Autodesk Fusion 360 part; units mm, degrees
(part 10 of 25)
  arc A1461 (56.8014, 41.9498) -> (56.508, 41.8283) centre (56.6547, 41.889) ccw
  line L369 (50.6695, 43.3959) -> (50.1845, 43.3959)
  line L370 (59.69, 41.0137) -> (59.96, 40.7437)
  arc A1462 (39.2664, 37.5968) -> (39.0418, 37.3723) centre (39.1541, 37.4846) ccw
  line L371 (42.1259, 37.4845) -> (42.1259, 37.9695)
  line L372 (52.2859, 41.2945) -> (52.2859, 41.7795)
  arc A1463 (50.9305, 40.5829) -> (50.9305, 40.2654) centre (50.9305, 40.4241) ccw
  arc A1464 (52.6557, 41.9247) -> (52.4312, 42.1493) centre (52.5434, 42.037) ccw
  arc A1465 (57.3078, 40.6314) -> (57.5323, 40.8559) centre (57.4201, 40.7437) ccw
  arc A1466 (43.5851, 43.6309) -> (43.5851, 43.3134) centre (43.5851, 43.4721) ccw
  line L373 (43.6534, 39.497) -> (49.7574, 39.497)
  arc A1467 (41.2555, 36.4554) -> (41.2555, 36.7728) centre (41.2555, 36.6141) ccw
  arc A1468 (39.9123, 36.5018) -> (40.1368, 36.7264) centre (40.0246, 36.6141) ccw
  line L374 (59.42, 40.7437) -> (59.69, 41.0137)
  arc A1469 (42.2846, 37.9695) -> (41.9671, 37.9695) centre (42.1258, 37.9695) ccw
  arc A1470 (58.0081, 40.3282) -> (58.1296, 40.6216) centre (58.0689, 40.4749) ccw
  line L375 (42.1259, 41.2945) -> (42.1259, 42.0129)
  arc A1471 (43.0134, 41.6363) -> (42.8919, 41.9297) centre (42.9527, 41.783) ccw
  line L376 (56.6547, 42.037) -> (56.6547, 41.8891)
  arc A1472 (56.7768, 41.1795) -> (57.0701, 41.301) centre (56.9235, 41.2403) ccw
  arc A1473 (43.6534, 39.6557) -> (43.6534, 39.3383) centre (43.6534, 39.497) ccw
  line L377 (50.499, 39.9925) -> (50.9305, 40.4241)
  arc A1474 (50.2382, 39.5243) -> (50.1167, 39.8177) centre (50.1775, 39.671) ccw
  arc A1475 (48.9443, 41.8953) -> (49.1688, 41.6707) centre (49.0566, 41.783) ccw
  line L378 (51.4155, 40.4241) -> (52.2859, 41.2945)
  line L379 (49.7574, 39.497) -> (50.1775, 39.671)
  arc A1476 (56.6547, 41.8783) -> (56.6547, 42.1957) centre (56.6547, 42.037) ccw
  arc A1477 (41.9671, 37.4845) -> (42.2846, 37.4845) centre (42.1258, 37.4845) ccw
  arc A1478 (59.4807, 40.597) -> (59.3592, 40.8903) centre (59.42, 40.7437) ccw
  arc A1479 (49.7574, 39.3383) -> (49.7574, 39.6557) centre (49.7574, 39.497) ccw
  arc A1480 (50.0652, 39.7833) -> (50.2897, 39.5588) centre (50.1775, 39.6711) ccw
  line L380 (49.0566, 41.783) -> (42.9526, 41.783)
  arc A1481 (33.6167, 36.6332) -> (33.6167, 36.3157) centre (33.6167, 36.4745) ccw
  arc A1482 (42.0988, 41.3997) -> (42.3233, 41.1752) centre (42.2111, 41.2874) ccw
  arc A1483 (34.8511, 36.5867) -> (35.0756, 36.3621) centre (34.9634, 36.4744) ccw
  arc A1484 (50.3867, 40.1048) -> (50.6112, 39.8803) centre (50.4989, 39.9926) ccw
  arc A1485 (52.3982, 41.1823) -> (52.1736, 41.4068) centre (52.2859, 41.2946) ccw
  arc A1486 (41.1432, 36.7264) -> (41.3677, 36.5018) centre (41.2554, 36.6141) ccw
  arc A1487 (51.4155, 40.2654) -> (51.4155, 40.5829) centre (51.4155, 40.4241) ccw
  arc A1488 (59.3077, 40.8559) -> (59.5322, 40.6314) centre (59.42, 40.7437) ccw
  arc A1489 (42.9526, 41.9417) -> (42.9526, 41.6242) centre (42.9526, 41.7829) ccw
  arc A1490 (42.0136, 38.0817) -> (42.2382, 37.8572) centre (42.1259, 37.9695) ccw
  arc A1491 (40.0245, 36.7728) -> (40.0245, 36.4554) centre (40.0245, 36.6141) ccw
  arc A1492 (37.0245, 36.9634) -> (37.0245, 37.2809) centre (37.0245, 37.1221) ccw
  line L381 (58.7711, 40.4749) -> (59.42, 40.7437)
  arc A1493 (58.7711, 40.3162) -> (58.7711, 40.6337) centre (58.7711, 40.475) ccw
  line L382 (50.1775, 39.671) -> (50.499, 39.9925)
  arc A1494 (49.2018, 42.6377) -> (49.4264, 42.4132) centre (49.3141, 42.5255) ccw
  line L383 (42.9526, 41.783) -> (42.5325, 41.609)
  line L384 (50.9305, 40.4241) -> (51.4155, 40.4241)
  line L385 (50.1845, 43.3959) -> (49.3141, 42.5255)
  line L386 (42.1259, 42.0129) -> (43.5851, 43.4721)
  line L387 (41.2555, 40.4241) -> (42.1259, 41.2945)
  arc A1495 (41.2555, 40.2654) -> (41.2555, 40.5829) centre (41.2555, 40.4241) ccw
  arc A1496 (49.1554, 42.0405) -> (49.4729, 42.0405) centre (49.3142, 42.0405) ccw
  line L388 (58.0689, 40.4749) -> (58.7711, 40.4749)
  arc A1497 (59.8023, 40.9014) -> (59.5777, 41.1259) centre (59.69, 41.0136) ccw
  arc A1498 (35.611, 37.2809) -> (35.611, 36.9634) centre (35.611, 37.1221) ccw
  arc A1499 (64.5607, 40.597) -> (64.4392, 40.8903) centre (64.4999, 40.7437) ccw
  arc A1500 (65.8812, 40.7289) -> (66.1987, 40.7289) centre (66.04, 40.7289) ccw
  arc A1501 (66.3448, 40.9171) -> (66.443, 40.6151) centre (66.3939, 40.7661) ccw
  arc A1502 (60.0208, 40.8903) -> (59.8993, 40.597) centre (59.9601, 40.7437) ccw
  arc A1503 (66.04, 40.5702) -> (66.04, 40.8877) centre (66.04, 40.7289) ccw
  arc A1504 (66.4187, 40.6093) -> (66.3691, 40.9229) centre (66.3939, 40.7661) ccw
  arc A1505 (63.1489, 40.6337) -> (63.1489, 40.3162) centre (63.1489, 40.475) ccw
  arc A1506 (62.3423, 40.9014) -> (62.1177, 41.1259) centre (62.23, 41.0137) ccw
  arc A1507 (66.1987, 43.18) -> (65.8812, 43.18) centre (66.04, 43.18) ccw
  arc A1508 (66.04, 43.0212) -> (66.04, 43.3387) centre (66.04, 43.18) ccw
  arc A1509 (57.4808, 40.8903) -> (57.3593, 40.597) centre (57.4201, 40.7437) ccw
  arc A1510 (63.7904, 40.6216) -> (63.9119, 40.3282) centre (63.8512, 40.4749) ccw
  arc A1511 (42.2382, 37.3723) -> (42.0136, 37.5968) centre (42.1259, 37.4845) ccw
  arc A1512 (50.6112, 39.8803) -> (50.3867, 40.1048) centre (50.4989, 39.9926) ccw
  arc A1513 (49.6966, 39.6437) -> (49.8181, 39.3503) centre (49.7574, 39.497) ccw
  arc A1514 (58.0689, 40.6337) -> (58.0689, 40.3162) centre (58.0689, 40.475) ccw
  line L389 (61.3111, 40.4749) -> (61.96, 40.7437)
  line L390 (52.2859, 41.7795) -> (52.5434, 42.037)
  line L391 (40.0245, 36.6141) -> (41.2555, 36.6141)
  line L392 (56.9235, 41.2402) -> (57.42, 40.7437)
  line L393 (62.23, 41.0137) -> (62.5, 40.7437)
  arc A1515 (56.8135, 42.037) -> (56.496, 42.037) centre (56.6547, 42.037) ccw
  arc A1516 (59.8023, 41.1259) -> (59.5777, 40.9014) centre (59.69, 41.0137) ccw
  line L394 (39.1541, 37.4845) -> (40.0245, 36.6141)
  arc A1517 (51.3032, 40.5364) -> (51.5277, 40.3118) centre (51.4154, 40.4241) ccw
  arc A1518 (65.3878, 40.6982) -> (65.5319, 40.9811) centre (65.4599, 40.8396) ccw
  arc A1519 (60.6089, 40.6337) -> (60.6089, 40.3162) centre (60.6089, 40.475) ccw
  line L395 (61.96, 40.7437) -> (62.23, 41.0137)
  line L396 (59.96, 40.7437) -> (60.6089, 40.4749)
  line L397 (65.6861, 40.7661) -> (65.9211, 40.7289)
  line L398 (66.04, 40.7289) -> (66.1589, 40.7289)
  line L399 (65.9211, 40.7289) -> (66.04, 40.7289)
  arc A1520 (52.1736, 41.8917) -> (52.3982, 41.6672) centre (52.2859, 41.7795) ccw
  arc A1521 (52.1271, 41.2945) -> (52.4446, 41.2945) centre (52.2858, 41.2945) ccw
  line L400 (52.5434, 42.037) -> (56.6547, 42.037)
  arc A1522 (62.5608, 40.8903) -> (62.4393, 40.597) centre (62.5001, 40.7437) ccw
  line L401 (60.6089, 40.4749) -> (61.3111, 40.4749)
  line L402 (56.6547, 41.8891) -> (56.9235, 41.2402)
  arc A1523 (59.8478, 40.6314) -> (60.0723, 40.8559) centre (59.9601, 40.7436) ccw
  arc A1524 (65.7109, 40.9229) -> (65.6613, 40.6093) centre (65.6861, 40.7661) ccw
  arc A1525 (66.04, 43.3387) -> (66.04, 43.0212) centre (66.04, 43.18) ccw
  arc A1526 (56.496, 41.8891) -> (56.8135, 41.8891) centre (56.6547, 41.8891) ccw
  arc A1527 (52.5434, 42.1957) -> (52.5434, 41.8783) centre (52.5434, 42.037) ccw
  line L403 (62.5, 40.7437) -> (63.1489, 40.4749)
  arc A1528 (65.9211, 40.8877) -> (65.9211, 40.5702) centre (65.9211, 40.7289) ccw
  arc A1529 (66.1988, 43.18) -> (65.8813, 43.18) centre (66.0401, 43.18) ccw
  line L404 (41.2555, 36.6141) -> (42.1259, 37.4845)
  arc A1530 (63.0881, 40.3282) -> (63.2096, 40.6216) centre (63.1489, 40.4749) ccw
  arc A1531 (60.5481, 40.3282) -> (60.6696, 40.6216) centre (60.6089, 40.4749) ccw
  line L405 (65.2479, 40.9476) -> (65.4599, 40.8396)
  arc A1532 (65.637, 40.6151) -> (65.7352, 40.9171) centre (65.6861, 40.7661) ccw
  arc A1533 (63.8511, 40.3162) -> (63.8511, 40.6337) centre (63.8511, 40.475) ccw
  arc A1534 (52.4446, 41.7795) -> (52.1271, 41.7795) centre (52.2858, 41.7795) ccw
  arc A1535 (65.8962, 40.5721) -> (65.9459, 40.8857) centre (65.9211, 40.7289) ccw
  arc A1536 (57.0357, 41.3525) -> (56.8112, 41.128) centre (56.9234, 41.2402) ccw
  arc A1537 (65.5089, 40.9906) -> (65.4108, 40.6886) centre (65.4599, 40.8396) ccw
  line L406 (42.1259, 37.9695) -> (43.6534, 39.497)
  arc A1538 (65.32, 41.0891) -> (65.1758, 40.8062) centre (65.2479, 40.9476) ccw
  arc A1539 (64.3877, 40.8559) -> (64.6122, 40.6314) centre (64.5, 40.7437) ccw
  line L407 (63.1489, 40.4749) -> (63.8511, 40.4749)
  arc A1540 (65.1488, 41.2159) -> (64.9621, 40.959) centre (65.0555, 41.0874) ccw
  arc A1541 (65.8813, 40.7289) -> (66.1988, 40.7289) centre (66.0401, 40.7289) ccw
  line L408 (64.9496, 41.1933) -> (65.0555, 41.0874)
  arc A1542 (66.04, 40.8877) -> (66.04, 40.5702) centre (66.04, 40.7289) ccw
  arc A1543 (66.3691, 45.4371) -> (66.4187, 45.7507) centre (66.3939, 45.5939) ccw
  arc A1544 (66.04, 43.3387) -> (66.04, 43.0212) centre (66.04, 43.18) ccw
  arc A1545 (67.5513, 43.0213) -> (67.5513, 43.3388) centre (67.5513, 43.1801) ccw
  arc A1546 (66.1988, 43.18) -> (65.8813, 43.18) centre (66.0401, 43.18) ccw
  arc A1547 (66.7388, 41.076) -> (66.9254, 40.8192) centre (66.8321, 40.9476) ccw
  arc A1548 (61.3111, 40.3162) -> (61.3111, 40.6337) centre (61.3111, 40.475) ccw
  line L409 (66.04, 43.18) -> (66.04, 40.7289)
  arc A1549 (66.6692, 40.6886) -> (66.5711, 40.9906) centre (66.6201, 40.8396) ccw
  line L410 (66.1589, 40.7289) -> (66.3939, 40.7661)
  line L411 (65.0555, 41.0874) -> (65.2479, 40.9476)
  arc A1550 (62.3423, 41.1259) -> (62.1177, 40.9014) centre (62.23, 41.0136) ccw
  arc A1551 (62.0207, 40.597) -> (61.8992, 40.8903) centre (61.96, 40.7437) ccw
  arc A1552 (67.3945, 44.2139) -> (67.7081, 44.2636) centre (67.5513, 44.2388) ccw
  arc A1553 (66.5711, 45.3694) -> (66.6692, 45.6714) centre (66.6201, 45.5204) ccw
  line L412 (66.6201, 40.8396) -> (66.8321, 40.9476)
  arc A1554 (66.76, 45.2709) -> (66.9042, 45.5538) centre (66.8321, 45.4124) ccw
  arc A1555 (65.0619, 41.3055) -> (64.8373, 41.081) centre (64.9496, 41.1932) ccw
  line L413 (66.1589, 45.6311) -> (66.04, 45.6311)
  arc A1556 (67.3925, 43.18) -> (67.71, 43.18) centre (67.5513, 43.18) ccw
  arc A1557 (67.6651, 41.8372) -> (67.3631, 41.9354) centre (67.5141, 41.8863) ccw
  line L414 (67.3326, 44.9119) -> (67.1928, 45.1043)
  line L415 (67.5141, 41.8863) -> (67.5513, 42.1213)
  line L416 (67.1928, 41.2557) -> (67.3326, 41.4481)
  line L417 (67.5141, 44.4737) -> (67.4406, 44.6999)
  arc A1558 (67.0643, 41.349) -> (67.3212, 41.1623) centre (67.1928, 41.2557) ccw
  arc A1559 (66.1838, 45.7879) -> (66.1341, 45.4743) centre (66.159, 45.6311) ccw
  arc A1560 (67.305, 41.1434) -> (67.0805, 41.3679) centre (67.1927, 41.2556) ccw
  arc A1561 (67.71, 43.18) -> (67.3925, 43.18) centre (67.5513, 43.18) ccw
  arc A1562 (67.5916, 44.749) -> (67.2896, 44.6509) centre (67.4406, 44.7) ccw
  arc A1563 (67.1179, 40.959) -> (66.9312, 41.2159) centre (67.0246, 41.0875) ccw
  line L418 (65.4599, 40.8396) -> (65.6861, 40.7661)
  line L419 (67.5513, 43.18) -> (66.04, 43.18)
  arc A1564 (66.04, 45.7898) -> (66.04, 45.4723) centre (66.04, 45.6311) ccw
  arc A1565 (67.6709, 44.4985) -> (67.3573, 44.4489) centre (67.5141, 44.4737) ccw
  line L420 (67.5513, 44.2387) -> (67.5141, 44.4737)
  arc A1566 (66.443, 45.7449) -> (66.3448, 45.4429) centre (66.3939, 45.5939) ccw
  line L421 (67.4406, 44.6999) -> (67.3326, 44.9119)
  line L422 (67.3326, 41.4481) -> (67.4406, 41.6601)
  arc A1567 (67.1911, 41.5202) -> (67.474, 41.376) centre (67.3326, 41.4481) ccw
  arc A1568 (61.2504, 40.6216) -> (61.3719, 40.3282) centre (61.3111, 40.4749) ccw
  line L423 (66.04, 40.7289) -> (66.04, 43.18)
  line L424 (63.8511, 40.4749) -> (64.5, 40.7437)
  arc A1569 (66.9312, 45.1441) -> (67.1179, 45.401) centre (67.0245, 45.2726) ccw
  arc A1570 (66.9254, 45.5408) -> (66.7388, 45.2839) centre (66.8321, 45.4124) ccw
  line L425 (67.5513, 43.18) -> (67.5513, 44.2387)
  arc A1571 (67.71, 44.2387) -> (67.3925, 44.2387) centre (67.5513, 44.2387) ccw
  arc A1572 (66.1341, 40.8857) -> (66.1838, 40.5721) centre (66.159, 40.7289) ccw
  arc A1573 (66.9042, 40.8062) -> (66.76, 41.0891) centre (66.8321, 40.9476) ccw
  arc A1574 (65.0619, 41.081) -> (64.8373, 41.3055) centre (64.9496, 41.1932) ccw
  line L426 (66.3939, 45.5939) -> (66.1589, 45.6311)
  arc A1575 (66.9123, 41.1997) -> (67.1368, 40.9752) centre (67.0246, 41.0875) ccw
  arc A1576 (67.582, 41.588) -> (67.2991, 41.7321) centre (67.4406, 41.66) ccw
  line L427 (64.5, 40.7437) -> (64.9496, 41.1933)
  arc A1577 (67.2991, 44.6279) -> (67.582, 44.772) centre (67.4406, 44.7) ccw
  line L428 (66.3939, 40.7661) -> (66.6201, 40.8396)
  arc A1578 (61.8477, 40.8559) -> (62.0722, 40.6314) centre (61.9599, 40.7437) ccw
  arc A1579 (66.1589, 40.5702) -> (66.1589, 40.8877) centre (66.1589, 40.7289) ccw
  line L429 (66.6201, 45.5204) -> (66.3939, 45.5939)
  line L430 (66.8321, 45.4124) -> (66.6201, 45.5204)
  arc A1580 (65.1546, 40.8192) -> (65.3412, 41.076) centre (65.2479, 40.9476) ccw
  arc A1581 (64.9432, 40.9752) -> (65.1677, 41.1997) centre (65.0555, 41.0874) ccw
  arc A1582 (62.3878, 40.6314) -> (62.6123, 40.8559) centre (62.5001, 40.7437) ccw
  arc A1583 (67.2896, 41.7091) -> (67.5916, 41.611) centre (67.4406, 41.66) ccw
  arc A1584 (67.461, 41.3548) -> (67.2041, 41.5414) centre (67.3325, 41.4481) ccw
  line L431 (64.5, 45.6163) -> (63.8511, 45.8851)
  arc A1585 (66.1988, 45.6311) -> (65.8813, 45.6311) centre (66.0401, 45.6311) ccw
  line L432 (65.9211, 45.6311) -> (65.6861, 45.5939)
  arc A1586 (67.0805, 44.9921) -> (67.305, 45.2166) centre (67.1927, 45.1044) ccw
  arc A1587 (65.9459, 45.4743) -> (65.8962, 45.7879) centre (65.9211, 45.6311) ccw
  arc A1588 (62.6123, 45.5041) -> (62.3878, 45.7286) centre (62.5001, 45.6164) ccw
  arc A1589 (67.2041, 44.8186) -> (67.461, 45.0052) centre (67.3325, 44.9119) ccw
  arc A1590 (63.1489, 46.0438) -> (63.1489, 45.7263) centre (63.1489, 45.8851) ccw
  arc A1591 (61.9986, 45.7722) -> (61.8772, 45.4788) centre (61.9379, 45.6255) ccw
  arc A1592 (67.474, 44.984) -> (67.1911, 44.8398) centre (67.3326, 44.9119) ccw
  arc A1593 (61.7791, 45.6255) -> (62.0966, 45.6255) centre (61.9379, 45.6255) ccw
  arc A1594 (67.3925, 42.1213) -> (67.71, 42.1213) centre (67.5513, 42.1213) ccw
  arc A1595 (61.9357, 46.3347) -> (61.6424, 46.2132) centre (61.7891, 46.2739) ccw
  arc A1596 (63.9119, 46.0318) -> (63.7904, 45.7384) centre (63.8512, 45.8851) ccw
  line L433 (65.0555, 45.2726) -> (64.9496, 45.1667)
  arc A1597 (66.04, 45.4723) -> (66.04, 45.7898) centre (66.04, 45.6311) ccw
  line L434 (63.8511, 45.8851) -> (63.1489, 45.8851)
  line L435 (67.0245, 45.2726) -> (66.8321, 45.4124)
  line L436 (60.2439, 47.819) -> (59.8845, 47.9679)
  line L437 (66.04, 43.18) -> (67.5513, 43.18)
  arc A1598 (64.8373, 45.279) -> (65.0619, 45.0544) centre (64.9496, 45.1667) ccw
  line L438 (63.1489, 45.8851) -> (62.5, 45.6163)
  arc A1599 (65.6613, 45.7507) -> (65.7109, 45.4371) centre (65.6861, 45.5939) ccw
  arc A1600 (64.4392, 45.4697) -> (64.5607, 45.763) centre (64.4999, 45.6163) ccw
  arc A1601 (66.04, 43.3388) -> (66.04, 43.0213) centre (66.04, 43.1801) ccw
  line L439 (67.4406, 41.6601) -> (67.5141, 41.8863)
  arc A1602 (67.3573, 41.9111) -> (67.6709, 41.8615) centre (67.5141, 41.8863) ccw
  line L440 (67.5513, 42.1213) -> (67.5513, 43.18)
  line L441 (67.1928, 45.1043) -> (67.0245, 45.2726)
  line L442 (61.789, 46.2739) -> (60.519, 47.5439)
  arc A1603 (60.4068, 47.4317) -> (60.6313, 47.6562) centre (60.5191, 47.544) ccw
  arc A1604 (64.8373, 45.0544) -> (65.0619, 45.279) centre (64.9496, 45.1667) ccw
  arc A1605 (60.3562, 47.9313) -> (60.1317, 47.7068) centre (60.2439, 47.8191) ccw
  line L443 (65.2479, 45.4124) -> (65.0555, 45.2726)
  line L444 (64.9496, 45.1667) -> (64.5, 45.6163)
  arc A1606 (65.5319, 45.3789) -> (65.3878, 45.6618) centre (65.4599, 45.5204) ccw
  line L445 (67.0245, 41.0874) -> (67.1928, 41.2557)
  arc A1607 (66.5481, 40.9811) -> (66.6922, 40.6982) centre (66.6202, 40.8396) ccw
  arc A1608 (62.0966, 45.9145) -> (61.7791, 45.9145) centre (61.9379, 45.9145) ccw
  arc A1609 (67.3212, 45.1977) -> (67.0643, 45.011) centre (67.1928, 45.1044) ccw
  arc A1610 (59.9453, 48.1146) -> (59.8238, 47.8212) centre (59.8846, 47.9679) ccw
  line L446 (59.8845, 47.9679) -> (59.2617, 47.9679)
  arc A1611 (66.6922, 45.6618) -> (66.5481, 45.3789) centre (66.6201, 45.5204) ccw
  arc A1612 (60.1832, 47.6724) -> (60.3047, 47.9657) centre (60.2439, 47.8191) ccw
  arc A1613 (65.8813, 43.18) -> (66.1988, 43.18) centre (66.0401, 43.18) ccw
  arc A1614 (65.1677, 45.1603) -> (64.9432, 45.3848) centre (65.0555, 45.2726) ccw
  line L447 (60.519, 47.5439) -> (60.2439, 47.819)
  arc A1615 (61.8992, 45.4697) -> (62.0207, 45.763) centre (61.96, 45.6163) ccw
  line L448 (62.23, 45.3463) -> (61.96, 45.6163)
  arc A1616 (62.4393, 45.763) -> (62.5608, 45.4697) centre (62.5001, 45.6164) ccw
  line L449 (65.4599, 45.5204) -> (65.2479, 45.4124)
  arc A1617 (65.4108, 45.6714) -> (65.5089, 45.3694) centre (65.4598, 45.5204) ccw
  arc A1618 (61.7912, 45.8538) -> (62.0846, 45.9753) centre (61.9379, 45.9145) ccw
  arc A1619 (67.7081, 42.0964) -> (67.3945, 42.1461) centre (67.5513, 42.1212) ccw
  arc A1620 (64.9621, 45.401) -> (65.1488, 45.1441) centre (65.0555, 45.2726) ccw
  arc A1621 (67.3631, 44.4246) -> (67.6651, 44.5228) centre (67.5141, 44.4737) ccw
  line L450 (66.8321, 40.9476) -> (67.0245, 41.0874)
  arc A1622 (66.04, 43.0213) -> (66.04, 43.3388) centre (66.04, 43.1801) ccw
  arc A1623 (65.1758, 45.5538) -> (65.32, 45.2709) centre (65.2479, 45.4124) ccw
  line L451 (65.6861, 45.5939) -> (65.4599, 45.5204)
  arc A1624 (67.1368, 45.3848) -> (66.9123, 45.1603) centre (67.0246, 45.2726) ccw
  arc A1625 (63.8511, 45.7263) -> (63.8511, 46.0438) centre (63.8511, 45.8851) ccw
  arc A1626 (67.5513, 43.0212) -> (67.5513, 43.3387) centre (67.5513, 43.18) ccw
  arc A1627 (66.1987, 45.6311) -> (65.8812, 45.6311) centre (66.04, 45.6311) ccw
  line L452 (60.6089, 47.7647) -> (61.3111, 47.7647)
  arc A1628 (62.872, 49.1181) -> (62.5786, 49.2396) centre (62.7253, 49.1788) ccw
  line L453 (61.9379, 45.6255) -> (61.9379, 45.9145)
  line L454 (61.9379, 45.9145) -> (61.789, 46.2739)
  arc A1629 (65.8812, 43.18) -> (66.1987, 43.18) centre (66.04, 43.18) ccw
  line L455 (66.04, 45.6311) -> (65.9211, 45.6311)
  arc A1630 (58.8319, 51.442) -> (58.7104, 51.1486) centre (58.7711, 51.2953) ccw
  arc A1631 (57.3593, 51.1732) -> (57.4808, 50.8799) centre (57.42, 51.0266) ccw
  line L456 (61.3111, 51.2953) -> (60.6089, 51.2953)
  line L457 (61.3111, 47.7647) -> (61.96, 48.0335)
  arc A1632 (61.8477, 48.1457) -> (62.0722, 47.9212) centre (61.9599, 48.0335) ccw
  arc A1633 (62.5786, 49.8204) -> (62.872, 49.9419) centre (62.7253, 49.8812) ccw
  arc A1634 (65.7352, 45.4429) -> (65.637, 45.7449) centre (65.6861, 45.5939) ccw
  arc A1635 (59.5777, 50.8688) -> (59.8023, 50.6443) centre (59.69, 50.7566) ccw
  arc A1636 (62.0207, 47.8868) -> (61.8992, 48.1801) centre (61.9599, 48.0334) ccw
  arc A1637 (62.6032, 50.5907) -> (62.3099, 50.4692) centre (62.4566, 50.5299) ccw
  line L458 (61.96, 48.0335) -> (62.4565, 48.53)
  line L459 (66.04, 45.6311) -> (66.04, 43.18)
  arc A1638 (65.3412, 45.2839) -> (65.1546, 45.5408) centre (65.2479, 45.4124) ccw
  line L460 (57.15, 50.7565) -> (56.88, 51.0265)
  arc A1639 (62.5665, 49.1789) -> (62.884, 49.1789) centre (62.7253, 49.1789) ccw
  arc A1640 (60.0208, 48.1801) -> (59.8993, 47.8868) centre (59.96, 48.0335) ccw
  arc A1641 (59.8023, 48.1912) -> (59.5777, 48.4157) centre (59.69, 48.3035) ccw
  line L461 (59.2617, 47.9679) -> (59.42, 48.0335)
  arc A1642 (62.0722, 45.7286) -> (61.8477, 45.5041) centre (61.9599, 45.6164) ccw
  line L462 (61.96, 45.6163) -> (61.9379, 45.6255)
  line L463 (66.04, 43.18) -> (66.04, 45.6311)
  arc A1643 (59.5322, 51.1388) -> (59.3077, 50.9143) centre (59.42, 51.0266) ccw
  arc A1644 (59.8478, 47.9212) -> (60.0723, 48.1457) centre (59.9601, 48.0334) ccw
  arc A1645 (60.6313, 47.6562) -> (60.4068, 47.4317) centre (60.5191, 47.5439) ccw
  arc A1646 (59.3077, 48.1457) -> (59.5322, 47.9212) centre (59.42, 48.0335) ccw
  arc A1647 (62.1177, 45.2341) -> (62.3423, 45.4586) centre (62.23, 45.3464) ccw
  arc A1648 (61.6768, 46.1617) -> (61.9013, 46.3862) centre (61.7891, 46.2739) ccw
  arc A1649 (60.6089, 47.9235) -> (60.6089, 47.606) centre (60.6089, 47.7648) ccw
  line L464 (58.7711, 51.2953) -> (58.0689, 51.2953)
  arc A1650 (57.5323, 50.9143) -> (57.3078, 51.1388) centre (57.4201, 51.0266) ccw
  line L465 (62.5, 45.6163) -> (62.23, 45.3463)
  arc A1651 (65.9211, 45.7898) -> (65.9211, 45.4723) centre (65.9211, 45.6311) ccw
  arc A1652 (59.8845, 47.8091) -> (59.8845, 48.1266) centre (59.8845, 47.9679) ccw
  arc A1653 (59.3592, 50.8799) -> (59.4807, 51.1732) centre (59.42, 51.0266) ccw
  arc A1654 (58.1296, 51.1486) -> (58.0081, 51.442) centre (58.0689, 51.2953) ccw
  arc A1655 (62.0722, 51.1388) -> (61.8477, 50.9143) centre (61.9599, 51.0266) ccw
  arc A1656 (66.1589, 45.4723) -> (66.1589, 45.7898) centre (66.1589, 45.6311) ccw
  line L466 (59.69, 50.7565) -> (59.42, 51.0265)
  line L467 (62.7253, 49.1789) -> (62.7253, 49.8811)
  arc A1657 (56.9922, 51.1388) -> (56.7677, 50.9143) centre (56.88, 51.0266) ccw
  arc A1658 (63.2096, 45.7384) -> (63.0881, 46.0318) centre (63.1488, 45.8851) ccw
  arc A1659 (60.5481, 47.618) -> (60.6696, 47.9114) centre (60.6089, 47.7647) ccw
  arc A1660 (64.6122, 45.7286) -> (64.3877, 45.5041) centre (64.4999, 45.6163) ccw
  arc A1661 (62.5688, 48.4178) -> (62.3443, 48.6423) centre (62.4565, 48.53) ccw
  arc A1662 (62.1177, 45.4586) -> (62.3423, 45.2341) centre (62.23, 45.3464) ccw
  arc A1663 (65.8813, 43.18) -> (66.1988, 43.18) centre (66.0401, 43.18) ccw
  line L468 (57.42, 51.0265) -> (57.15, 50.7565)
  arc A1664 (57.0377, 50.8688) -> (57.2623, 50.6443) centre (57.15, 50.7566) ccw
  arc A1665 (66.04, 43.3388) -> (66.04, 43.0213) centre (66.04, 43.1801) ccw
  arc A1666 (61.3111, 51.1365) -> (61.3111, 51.454) centre (61.3111, 51.2953) ccw
  arc A1667 (61.2504, 47.9114) -> (61.3719, 47.618) centre (61.3111, 47.7647) ccw
  line L469 (62.4565, 50.53) -> (61.96, 51.0265)
  arc A1668 (59.5777, 50.6443) -> (59.8023, 50.8688) centre (59.69, 50.7566) ccw
  line L470 (62.7253, 49.8811) -> (62.4565, 50.53)
  arc A1669 (60.6089, 51.454) -> (60.6089, 51.1365) centre (60.6089, 51.2953) ccw
  arc A1670 (58.0689, 51.454) -> (58.0689, 51.1365) centre (58.0689, 51.2953) ccw
  line L471 (58.0689, 51.2953) -> (57.42, 51.0265)
  line L472 (59.42, 48.0335) -> (59.69, 48.3035)
  line L473 (51.1511, 51.2953) -> (50.4489, 51.2953)
  arc A1671 (57.0377, 50.6443) -> (57.2623, 50.8688) centre (57.15, 50.7566) ccw
  arc A1672 (49.7393, 51.1732) -> (49.8608, 50.8799) centre (49.8, 51.0266) ccw
  arc A1673 (49.1992, 50.8799) -> (49.3207, 51.1732) centre (49.26, 51.0266) ccw
  arc A1674 (52.9889, 51.454) -> (52.9889, 51.1365) centre (52.9889, 51.2953) ccw
  line L474 (59.96, 51.0265) -> (59.69, 50.7565)
  arc A1675 (52.4523, 50.9143) -> (52.2278, 51.1388) centre (52.34, 51.0266) ccw
  arc A1676 (61.3111, 47.606) -> (61.3111, 47.9235) centre (61.3111, 47.7648) ccw
  arc A1677 (59.2617, 48.1266) -> (59.2617, 47.8091) centre (59.2617, 47.9679) ccw
  arc A1678 (59.4807, 47.8868) -> (59.3592, 48.1801) centre (59.42, 48.0335) ccw
  arc A1679 (59.8993, 51.1732) -> (60.0208, 50.8799) centre (59.9601, 51.0266) ccw
  line L475 (59.96, 48.0335) -> (60.6089, 47.7647)
  arc A1680 (61.8992, 50.8799) -> (62.0207, 51.1732) centre (61.9599, 51.0266) ccw
  line L476 (59.42, 51.0265) -> (58.7711, 51.2953)
  line L477 (52.9889, 51.2953) -> (52.34, 51.0265)
  line L478 (49.8, 51.0265) -> (49.53, 50.7565)
  line L479 (61.96, 51.0265) -> (61.3111, 51.2953)
  arc A1681 (47.9089, 51.454) -> (47.9089, 51.1365) centre (47.9089, 51.2953) ccw
  arc A1682 (55.5289, 51.454) -> (55.5289, 51.1365) centre (55.5289, 51.2953) ccw
  arc A1683 (62.884, 49.8811) -> (62.5665, 49.8811) centre (62.7253, 49.8811) ccw
  arc A1684 (51.9122, 51.1388) -> (51.6877, 50.9143) centre (51.7999, 51.0266) ccw
  line L480 (54.34, 51.0265) -> (53.6911, 51.2953)
  arc A1685 (54.2792, 50.8799) -> (54.4007, 51.1732) centre (54.34, 51.0266) ccw
  arc A1686 (61.3719, 51.442) -> (61.2504, 51.1486) centre (61.3112, 51.2953) ccw
  line L481 (60.6089, 51.2953) -> (59.96, 51.0265)
  arc A1687 (46.8322, 51.1388) -> (46.6077, 50.9143) centre (46.72, 51.0266) ccw
  arc A1688 (54.4977, 50.8688) -> (54.7223, 50.6443) centre (54.61, 50.7566) ccw
  arc A1689 (51.1511, 51.1365) -> (51.1511, 51.454) centre (51.1511, 51.2953) ccw
  arc A1690 (52.2793, 51.1732) -> (52.4008, 50.8799) centre (52.3401, 51.0266) ccw
  line L482 (56.2311, 51.2953) -> (55.5289, 51.2953)
  line L483 (54.61, 50.7565) -> (54.34, 51.0265)
  arc A1691 (46.6592, 50.8799) -> (46.7807, 51.1732) centre (46.72, 51.0265) ccw
  arc A1692 (47.3723, 50.9143) -> (47.1478, 51.1388) centre (47.2601, 51.0266) ccw
  line L484 (51.8, 51.0265) -> (51.1511, 51.2953)
  arc A1693 (54.4522, 51.1388) -> (54.2277, 50.9143) centre (54.3399, 51.0266) ccw
  line L485 (50.4489, 51.2953) -> (49.8, 51.0265)
  arc A1694 (46.8777, 50.8688) -> (47.1023, 50.6443) centre (46.99, 50.7566) ccw
  arc A1695 (46.8777, 50.6443) -> (47.1023, 50.8688) centre (46.99, 50.7566) ccw
  arc A1696 (56.2919, 51.442) -> (56.1704, 51.1486) centre (56.2311, 51.2953) ccw
  line L486 (59.69, 48.3035) -> (59.96, 48.0335)
  arc A1697 (59.2009, 48.1146) -> (59.3224, 47.8212) centre (59.2616, 47.9679) ccw
  arc A1698 (58.7711, 51.1365) -> (58.7711, 51.454) centre (58.7711, 51.2953) ccw
  line L487 (49.53, 50.7565) -> (49.26, 51.0265)
  line L488 (46.72, 51.0265) -> (46.0711, 51.2953)
  line L489 (49.26, 51.0265) -> (48.6111, 51.2953)
  arc A1699 (54.4977, 50.6443) -> (54.7223, 50.8688) centre (54.61, 50.7566) ccw
  arc A1700 (60.0723, 50.9143) -> (59.8478, 51.1388) centre (59.9601, 51.0266) ccw
  line L490 (53.6911, 51.2953) -> (52.9889, 51.2953)
  arc A1701 (62.3099, 48.5908) -> (62.6032, 48.4693) centre (62.4566, 48.5301) ccw
  arc A1702 (54.8193, 51.1732) -> (54.9408, 50.8799) centre (54.8801, 51.0266) ccw
  arc A1703 (46.1319, 51.442) -> (46.0104, 51.1486) centre (46.0712, 51.2953) ccw
  arc A1704 (56.2311, 51.1365) -> (56.2311, 51.454) centre (56.2311, 51.2953) ccw
  line L491 (62.4565, 48.53) -> (62.7253, 49.1789)
  arc A1705 (54.9923, 50.9143) -> (54.7678, 51.1388) centre (54.8801, 51.0266) ccw
  arc A1706 (62.3443, 50.4177) -> (62.5688, 50.6422) centre (62.4566, 50.53) ccw
  line L492 (46.99, 50.7565) -> (46.72, 51.0265)
  line L493 (47.9089, 51.2953) -> (47.26, 51.0265)
  arc A1707 (55.5896, 51.1486) -> (55.4681, 51.442) centre (55.5289, 51.2953) ccw
  arc A1708 (51.2119, 51.442) -> (51.0904, 51.1486) centre (51.1512, 51.2953) ccw
  arc A1709 (50.4489, 51.454) -> (50.4489, 51.1365) centre (50.4489, 51.2953) ccw
  arc A1710 (60.6696, 51.1486) -> (60.5481, 51.442) centre (60.6089, 51.2953) ccw
  arc A1711 (59.8023, 48.4157) -> (59.5777, 48.1912) centre (59.69, 48.3035) ccw
  arc A1712 (51.9577, 50.6443) -> (52.1823, 50.8688) centre (52.07, 50.7566) ccw
  arc A1713 (53.7519, 51.442) -> (53.6304, 51.1486) centre (53.6912, 51.2953) ccw
  arc A1714 (42.2923, 50.9143) -> (42.0678, 51.1388) centre (42.18, 51.0266) ccw
  line L494 (54.88, 51.0265) -> (54.61, 50.7565)
  arc A1715 (47.1993, 51.1732) -> (47.3208, 50.8799) centre (47.26, 51.0266) ccw
  arc A1716 (41.7977, 50.6443) -> (42.0223, 50.8688) centre (41.91, 50.7566) ccw
  arc A1717 (53.6911, 51.1365) -> (53.6911, 51.454) centre (53.6911, 51.2953) ccw
  line L495 (47.26, 51.0265) -> (46.99, 50.7565)
  arc A1718 (49.4177, 50.6443) -> (49.6423, 50.8688) centre (49.53, 50.7566) ccw
  line L496 (45.3689, 51.2953) -> (44.72, 51.0265)
  arc A1719 (51.7392, 50.8799) -> (51.8607, 51.1732) centre (51.7999, 51.0266) ccw
  line L497 (43.5311, 51.2953) -> (42.8289, 51.2953)
  arc A1720 (36.4992, 50.8799) -> (36.6207, 51.1732) centre (36.56, 51.0266) ccw
  arc A1721 (43.5311, 51.1365) -> (43.5311, 51.454) centre (43.5311, 51.2953) ccw
  line L498 (37.7489, 51.2953) -> (37.1, 51.0265)
  line L499 (35.9111, 51.2953) -> (35.2089, 51.2953)
  arc A1722 (37.0393, 51.1732) -> (37.1608, 50.8799) centre (37.1, 51.0266) ccw
  arc A1723 (37.2123, 50.9143) -> (36.9878, 51.1388) centre (37.1001, 51.0266) ccw
  arc A1724 (48.6719, 51.442) -> (48.5504, 51.1486) centre (48.6112, 51.2953) ccw
  arc A1725 (51.9577, 50.8688) -> (52.1823, 50.6443) centre (52.07, 50.7566) ccw
  line L500 (37.1, 51.0265) -> (36.83, 50.7565)
  line L501 (39.64, 51.0265) -> (39.37, 50.7565)
  arc A1726 (36.6722, 51.1388) -> (36.4477, 50.9143) centre (36.56, 51.0266) ccw
  line L502 (55.5289, 51.2953) -> (54.88, 51.0265)
  arc A1727 (38.5119, 51.442) -> (38.3904, 51.1486) centre (38.4511, 51.2953) ccw
  arc A1728 (35.9719, 51.442) -> (35.8504, 51.1486) centre (35.9112, 51.2953) ccw
  line L503 (56.88, 51.0265) -> (56.2311, 51.2953)
  arc A1729 (50.5096, 51.1486) -> (50.3881, 51.442) centre (50.4489, 51.2953) ccw
  arc A1730 (49.3722, 51.1388) -> (49.1477, 50.9143) centre (49.26, 51.0266) ccw
  arc A1731 (56.8192, 50.8799) -> (56.9407, 51.1732) centre (56.88, 51.0266) ccw
  arc A1732 (47.9696, 51.1486) -> (47.8481, 51.442) centre (47.9089, 51.2953) ccw
  arc A1733 (36.7177, 50.8688) -> (36.9423, 50.6443) centre (36.83, 50.7566) ccw
  line L504 (48.6111, 51.2953) -> (47.9089, 51.2953)
  line L505 (36.83, 50.7565) -> (36.56, 51.0265)
  line L506 (46.0711, 51.2953) -> (45.3689, 51.2953)
  line L507 (44.72, 51.0265) -> (44.45, 50.7565)
  arc A1734 (41.7522, 51.1388) -> (41.5277, 50.9143) centre (41.6399, 51.0266) ccw
  arc A1735 (38.4511, 51.1365) -> (38.4511, 51.454) centre (38.4511, 51.2953) ccw
  arc A1736 (37.8096, 51.1486) -> (37.6881, 51.442) centre (37.7489, 51.2953) ccw
  arc A1737 (53.0496, 51.1486) -> (52.9281, 51.442) centre (52.9888, 51.2953) ccw
  line L508 (52.07, 50.7565) -> (51.8, 51.0265)
  arc A1738 (36.7177, 50.6443) -> (36.9423, 50.8688) centre (36.83, 50.7566) ccw
  arc A1739 (44.3377, 50.6443) -> (44.5623, 50.8688) centre (44.45, 50.7566) ccw
  line L509 (41.91, 50.7565) -> (41.64, 51.0265)
  arc A1740 (35.2089, 51.454) -> (35.2089, 51.1365) centre (35.2089, 51.2953) ccw
  arc A1741 (44.3377, 50.8688) -> (44.5623, 50.6443) centre (44.45, 50.7566) ccw
  arc A1742 (45.3689, 51.454) -> (45.3689, 51.1365) centre (45.3689, 51.2953) ccw
  arc A1743 (48.6111, 51.1365) -> (48.6111, 51.454) centre (48.6111, 51.2953) ccw
  arc A1744 (39.0392, 50.8799) -> (39.1607, 51.1732) centre (39.1, 51.0266) ccw
  arc A1745 (44.1192, 50.8799) -> (44.2407, 51.1732) centre (44.1799, 51.0266) ccw
  line L510 (42.8289, 51.2953) -> (42.18, 51.0265)
  line L511 (39.1, 51.0265) -> (38.4511, 51.2953)
  line L512 (35.2089, 51.2953) -> (34.56, 51.0265)
  arc A1746 (44.8323, 50.9143) -> (44.6078, 51.1388) centre (44.72, 51.0266) ccw
  arc A1747 (49.4177, 50.8688) -> (49.6423, 50.6443) centre (49.53, 50.7566) ccw
  arc A1748 (49.9123, 50.9143) -> (49.6878, 51.1388) centre (49.8, 51.0266) ccw
  arc A1749 (39.2577, 50.8688) -> (39.4823, 50.6443) centre (39.37, 50.7566) ccw
  line L513 (36.56, 51.0265) -> (35.9111, 51.2953)
  arc A1750 (42.8896, 51.1486) -> (42.7681, 51.442) centre (42.8289, 51.2953) ccw
  arc A1751 (44.6593, 51.1732) -> (44.7808, 50.8799) centre (44.7201, 51.0266) ccw
  arc A1752 (35.9111, 51.1365) -> (35.9111, 51.454) centre (35.9111, 51.2953) ccw
  arc A1753 (42.1193, 51.1732) -> (42.2408, 50.8799) centre (42.1801, 51.0266) ccw
  arc A1754 (41.0519, 51.442) -> (40.9304, 51.1486) centre (40.9912, 51.2953) ccw
  line L514 (52.34, 51.0265) -> (52.07, 50.7565)
  line L515 (44.45, 50.7565) -> (44.18, 51.0265)
  line L516 (38.4511, 51.2953) -> (37.7489, 51.2953)
  arc A1755 (31.5768, 50.795) -> (31.3523, 50.5705) centre (31.4645, 50.6827) ccw
  arc A1756 (30.48, 51.2) -> (30.48, 50.8825) centre (30.48, 51.0413) ccw
  arc A1757 (30.6238, 51.1981) -> (30.5741, 50.8845) centre (30.599, 51.0413) ccw
  arc A1758 (29.7812, 50.6941) -> (29.5946, 50.951) centre (29.6879, 50.8225) ccw
  arc A1759 (42.8289, 51.454) -> (42.8289, 51.1365) centre (42.8289, 51.2953) ccw
  arc A1760 (30.1752, 50.8531) -> (30.077, 51.1551) centre (30.1261, 51.0041) ccw
  arc A1761 (40.9911, 51.1365) -> (40.9911, 51.454) centre (40.9911, 51.2953) ccw
  arc A1762 (39.7523, 50.9143) -> (39.5278, 51.1388) centre (39.64, 51.0266) ccw
  arc A1763 (31.2, 50.6811) -> (31.3442, 50.964) centre (31.2721, 50.8226) ccw
  arc A1764 (32.7296, 51.1486) -> (32.6081, 51.442) centre (32.6689, 51.2953) ccw
  line L517 (31.5704, 50.5769) -> (31.4645, 50.6828)
  arc A1765 (30.5989, 50.8825) -> (30.5989, 51.2) centre (30.5989, 51.0413) ccw
  arc A1766 (30.48, 49.3713) -> (30.48, 49.6888) centre (30.48, 49.5301) ccw
  line L518 (32.6689, 51.2953) -> (32.02, 51.0265)
  line L519 (29.6879, 50.8226) -> (29.4955, 50.6828)
  arc A1767 (34.1322, 51.1388) -> (33.9077, 50.9143) centre (34.0199, 51.0266) ccw
  line L520 (31.4645, 50.6828) -> (31.2721, 50.8226)
  line L521 (31.2721, 50.8226) -> (31.0601, 50.9306)
  arc A1768 (29.215, 50.6268) -> (29.4395, 50.4023) centre (29.3273, 50.5146) ccw
  arc A1769 (30.8091, 50.8473) -> (30.8587, 51.1609) centre (30.8339, 51.0041) ccw
  line L522 (30.5989, 51.0413) -> (30.48, 51.0413)
  arc A1770 (32.1323, 50.9143) -> (31.9078, 51.1388) centre (32.0201, 51.0266) ccw
  arc A1771 (30.3213, 49.53) -> (30.6388, 49.53) centre (30.4801, 49.53) ccw
  arc A1772 (31.0111, 50.7796) -> (31.1092, 51.0816) centre (31.0602, 50.9306) ccw
  line L523 (29.4955, 50.6828) -> (29.3272, 50.5145)
  arc A1773 (29.4021, 50.8112) -> (29.5888, 50.5543) centre (29.4955, 50.6827) ccw
  line L524 (34.56, 51.0265) -> (34.29, 50.7565)
  line L525 (39.37, 50.7565) -> (39.1, 51.0265)
  arc A1774 (34.4993, 51.1732) -> (34.6208, 50.8799) centre (34.5601, 51.0266) ccw
  line L526 (30.3611, 51.0413) -> (30.1261, 51.0041)
  arc A1775 (29.9719, 50.7891) -> (29.8278, 51.072) centre (29.8999, 50.9306) ccw
  arc A1776 (40.2889, 51.454) -> (40.2889, 51.1365) centre (40.2889, 51.2953) ccw
  arc A1777 (31.4581, 50.6892) -> (31.6826, 50.4646) centre (31.5704, 50.5769) ccw
  arc A1778 (41.7977, 50.8688) -> (42.0223, 50.6443) centre (41.91, 50.7566) ccw
  line L527 (40.2889, 51.2953) -> (39.64, 51.0265)
  arc A1779 (37.7489, 51.454) -> (37.7489, 51.1365) centre (37.7489, 51.2953) ccw
  arc A1780 (39.2577, 50.6443) -> (39.4823, 50.8688) centre (39.37, 50.7566) ccw
  arc A1781 (31.9593, 51.1732) -> (32.0808, 50.8799) centre (32.0201, 51.0266) ccw
  line L528 (30.8339, 51.0041) -> (30.5989, 51.0413)
  arc A1782 (30.883, 51.1551) -> (30.7848, 50.8531) centre (30.8339, 51.0041) ccw
  arc A1783 (29.6158, 50.964) -> (29.76, 50.6811) centre (29.6879, 50.8225) ccw
  line L529 (41.64, 51.0265) -> (40.9911, 51.2953)
  arc A1784 (30.6388, 51.0413) -> (30.3213, 51.0413) centre (30.4801, 51.0413) ccw
  line L530 (34.29, 50.7565) -> (34.02, 51.0265)
  line L531 (42.18, 51.0265) -> (41.91, 50.7565)
  arc A1785 (31.3654, 50.951) -> (31.1788, 50.6941) centre (31.2721, 50.8225) ccw
  line L532 (30.48, 51.0413) -> (30.3611, 51.0413)
  arc A1786 (39.5793, 51.1732) -> (39.7008, 50.8799) centre (39.6401, 51.0266) ccw
  arc A1787 (46.0711, 51.1365) -> (46.0711, 51.454) centre (46.0711, 51.2953) ccw
  arc A1788 (30.3611, 51.2) -> (30.3611, 50.8825) centre (30.3611, 51.0413) ccw
  line L533 (44.18, 51.0265) -> (43.5311, 51.2953)
  line L534 (40.9911, 51.2953) -> (40.2889, 51.2953)
  arc A1789 (43.5919, 51.442) -> (43.4704, 51.1486) centre (43.5312, 51.2953) ccw
  arc A1790 (40.3496, 51.1486) -> (40.2281, 51.442) centre (40.2889, 51.2953) ccw
  line L535 (30.48, 49.53) -> (30.48, 51.0413)
  arc A1791 (29.6077, 50.5705) -> (29.3832, 50.795) centre (29.4954, 50.6827) ccw
  arc A1792 (41.5792, 50.8799) -> (41.7007, 51.1732) centre (41.6399, 51.0266) ccw
  arc A1793 (35.2696, 51.1486) -> (35.1481, 51.442) centre (35.2089, 51.2953) ccw
  arc A1794 (39.2122, 51.1388) -> (38.9877, 50.9143) centre (39.1, 51.0266) ccw
  arc A1795 (33.4319, 51.442) -> (33.3104, 51.1486) centre (33.3712, 51.2953) ccw
  arc A1796 (45.4296, 51.1486) -> (45.3081, 51.442) centre (45.3689, 51.2953) ccw
  arc A1797 (44.2922, 51.1388) -> (44.0677, 50.9143) centre (44.1799, 51.0266) ccw
  arc A1798 (34.1777, 50.6443) -> (34.4023, 50.8688) centre (34.29, 50.7565) ccw
  arc A1799 (33.3711, 51.1365) -> (33.3711, 51.454) centre (33.3711, 51.2953) ccw
  arc A1800 (26.7373, 50.4646) -> (26.9619, 50.6892) centre (26.8496, 50.5769) ccw
  arc A1801 (27.6352, 50.8531) -> (27.537, 51.1551) centre (27.5861, 51.0041) ccw
  arc A1802 (27.94, 49.3713) -> (27.94, 49.6888) centre (27.94, 49.5301) ccw
  arc A1803 (30.3859, 50.8845) -> (30.3362, 51.1981) centre (30.361, 51.0413) ccw
  line L536 (27.94, 51.0413) -> (27.8211, 51.0413)
  line L537 (32.02, 51.0265) -> (31.5704, 50.5769)
  arc A1804 (30.48, 49.6888) -> (30.48, 49.3713) centre (30.48, 49.5301) ccw
  line L538 (29.0928, 50.5145) -> (28.9245, 50.6828)
  arc A1805 (25.8119, 51.442) -> (25.6904, 51.1486) centre (25.7512, 51.2953) ccw
  arc A1806 (27.2412, 50.6941) -> (27.0546, 50.951) centre (27.1479, 50.8225) ccw
  arc A1807 (26.3392, 50.8799) -> (26.4607, 51.1732) centre (26.3999, 51.0266) ccw
  line L539 (25.7511, 51.2953) -> (25.0489, 51.2953)
  arc A1808 (32.6689, 51.454) -> (32.6689, 51.1365) centre (32.6689, 51.2953) ccw
  arc A1809 (25.0489, 51.454) -> (25.0489, 51.1365) centre (25.0489, 51.2953) ccw
  arc A1810 (23.9342, 50.7853) -> (24.1587, 50.5607) centre (24.0465, 50.673) ccw
  arc A1811 (28.66, 50.6811) -> (28.8042, 50.964) centre (28.7321, 50.8226) ccw
  arc A1812 (26.8621, 50.8112) -> (27.0488, 50.5543) centre (26.9554, 50.6827) ccw
  line L540 (31.0601, 50.9306) -> (30.8339, 51.0041)
  arc A1813 (29.8508, 51.0816) -> (29.9489, 50.7796) centre (29.8999, 50.9306) ccw
  line L541 (26.8496, 50.5769) -> (26.4, 51.0265)
  arc A1814 (29.0816, 50.2599) -> (29.3384, 50.4465) centre (29.21, 50.3532) ccw
  line L542 (25.0489, 51.2953) -> (24.4, 51.0265)
  arc A1815 (27.7813, 49.53) -> (28.0988, 49.53) centre (27.9401, 49.53) ccw
  line L543 (27.94, 49.53) -> (27.94, 51.0413)
  arc A1816 (34.1777, 50.8688) -> (34.4023, 50.6443) centre (34.29, 50.7566) ccw
  arc A1817 (30.6387, 51.0413) -> (30.3212, 51.0413) centre (30.48, 51.0413) ccw
  arc A1818 (30.3212, 49.53) -> (30.6387, 49.53) centre (30.48, 49.53) ccw
  arc A1819 (30.1013, 51.1609) -> (30.1509, 50.8473) centre (30.1261, 51.0041) ccw
  arc A1820 (27.0677, 50.5705) -> (26.8432, 50.795) centre (26.9554, 50.6827) ccw
  line L544 (27.94, 51.0413) -> (27.94, 49.53)
  arc A1821 (26.5122, 51.1388) -> (26.2877, 50.9143) centre (26.3999, 51.0266) ccw
  line L545 (27.5861, 51.0041) -> (27.3599, 50.9306)
  arc A1822 (28.0838, 51.1981) -> (28.0341, 50.8845) centre (28.0589, 51.0413) ccw
  line L546 (24.4, 51.0265) -> (24.0465, 50.673)
  arc A1823 (28.9805, 50.4023) -> (29.205, 50.6268) centre (29.0928, 50.5146) ccw
  line L547 (26.4, 51.0265) -> (25.7511, 51.2953)
  arc A1824 (31.4581, 50.4646) -> (31.6826, 50.6892) centre (31.5704, 50.5769) ccw
  arc A1825 (34.6723, 50.9143) -> (34.4478, 51.1388) centre (34.5601, 51.0266) ccw
  arc A1826 (24.3393, 51.1732) -> (24.4608, 50.8799) centre (24.4001, 51.0266) ccw
  line L548 (33.3711, 51.2953) -> (32.6689, 51.2953)
  arc A1827 (26.7373, 50.6892) -> (26.9619, 50.4646) centre (26.8496, 50.5769) ccw
  arc A1828 (25.1096, 51.1486) -> (24.9881, 51.442) centre (25.0489, 51.2953) ccw
  arc A1829 (31.1322, 51.072) -> (30.9881, 50.7891) centre (31.0602, 50.9306) ccw
  arc A1830 (27.0758, 50.964) -> (27.22, 50.6811) centre (27.1479, 50.8225) ccw
  arc A1831 (31.3712, 50.5543) -> (31.5579, 50.8112) centre (31.4646, 50.6827) ccw
  arc A1832 (27.4319, 50.7891) -> (27.2878, 51.072) centre (27.3599, 50.9306) ccw
  arc A1833 (28.5922, 51.072) -> (28.4481, 50.7891) centre (28.5202, 50.9306) ccw
  line L549 (28.9245, 50.6828) -> (28.7321, 50.8226)
  line L550 (26.9555, 50.6828) -> (26.8496, 50.5769)
  line L551 (28.2939, 51.0041) -> (28.0589, 51.0413)
  arc A1834 (27.94, 50.8825) -> (27.94, 51.2) centre (27.94, 51.0413) ccw
  line L552 (28.7321, 50.8226) -> (28.5201, 50.9306)
  arc A1835 (25.7511, 51.1365) -> (25.7511, 51.454) centre (25.7511, 51.2953) ccw
  arc A1836 (28.343, 51.1551) -> (28.2448, 50.8531) centre (28.2939, 51.0041) ccw
  line L553 (30.1261, 51.0041) -> (29.8999, 50.9306)
  arc A1837 (30.48, 50.8825) -> (30.48, 51.2) centre (30.48, 51.0413) ccw
  line L554 (30.48, 51.0413) -> (30.48, 49.53)
  arc A1838 (27.7812, 49.53) -> (28.0987, 49.53) centre (27.94, 49.53) ccw
  arc A1839 (28.8254, 50.951) -> (28.6388, 50.6941) centre (28.7321, 50.8225) ccw
  arc A1840 (29.0816, 50.4465) -> (29.3384, 50.2599) centre (29.21, 50.3532) ccw
  arc A1841 (33.9592, 50.8799) -> (34.0807, 51.1732) centre (34.02, 51.0266) ccw
  line L555 (29.8999, 50.9306) -> (29.6879, 50.8226)
  line L556 (34.02, 51.0265) -> (33.3711, 51.2953)
  arc A1842 (28.4711, 50.7796) -> (28.5692, 51.0816) centre (28.5202, 50.9306) ccw
  arc A1843 (19.2087, 51.9811) -> (18.8912, 51.9811) centre (19.05, 51.9811) ccw
  arc A1844 (22.0019, 52.3818) -> (21.8804, 52.0884) centre (21.9412, 52.2351) ccw
  line L557 (19.05, 49.53) -> (19.05, 51.9811)
  line L558 (23.3553, 50.8209) -> (23.0865, 51.4698)
  arc A1845 (18.4208, 52.0214) -> (18.5189, 51.7194) centre (18.4698, 51.8704) ccw
  arc A1846 (28.0987, 51.0413) -> (27.7812, 51.0413) centre (27.94, 51.0413) ccw
  arc A1847 (18.9559, 51.8243) -> (18.9062, 52.1379) centre (18.931, 51.9811) ccw
  line L559 (29.3272, 50.5145) -> (29.21, 50.3532)
  arc A1848 (23.3553, 50.8317) -> (23.3553, 50.5142) centre (23.3553, 50.673) ccw
  arc A1849 (28.0589, 50.8825) -> (28.0589, 51.2) centre (28.0589, 51.0413) ccw
  arc A1850 (29.0368, 50.795) -> (28.8123, 50.5705) centre (28.9245, 50.6827) ccw
  arc A1851 (29.2212, 50.6079) -> (28.9643, 50.4212) centre (29.0928, 50.5145) ccw
  arc A1852 (28.0988, 51.0413) -> (27.7813, 51.0413) centre (27.9401, 51.0413) ccw
  line L560 (23.3553, 50.673) -> (23.3553, 50.8209)
  arc A1853 (21.9411, 52.0763) -> (21.9411, 52.3938) centre (21.9411, 52.2351) ccw
  arc A1854 (20.7023, 51.8541) -> (20.4778, 52.0786) centre (20.5901, 51.9664) ccw
  arc A1855 (23.1965, 50.673) -> (23.514, 50.673) centre (23.3553, 50.673) ccw
  arc A1856 (19.05, 52.1398) -> (19.05, 51.8223) centre (19.05, 51.9811) ccw
  line L561 (20.0345, 51.6226) -> (19.8421, 51.7624)
  arc A1857 (27.8211, 51.2) -> (27.8211, 50.8825) centre (27.8211, 51.0413) ccw
  arc A1858 (19.05, 49.3713) -> (19.05, 49.6888) centre (19.05, 49.5301) ccw
  line L562 (21.9411, 52.2351) -> (21.2389, 52.2351)
  arc A1859 (21.2389, 52.3938) -> (21.2389, 52.0763) centre (21.2389, 52.2351) ccw
  arc A1860 (27.94, 51.2) -> (27.94, 50.8825) centre (27.94, 51.0413) ccw
  arc A1861 (27.94, 49.6888) -> (27.94, 49.3713) centre (27.94, 49.5301) ccw
  arc A1862 (20.5293, 52.113) -> (20.6508, 51.8197) centre (20.5901, 51.9664) ccw
  arc A1863 (20.1468, 51.7348) -> (19.9223, 51.5103) centre (20.0345, 51.6226) ccw
  arc A1864 (18.1858, 51.9038) -> (18.33, 51.6209) centre (18.2579, 51.7623) ccw
  arc A1865 (18.5419, 51.7289) -> (18.3978, 52.0118) centre (18.4699, 51.8704) ccw
  arc A1866 (20.0281, 51.629) -> (20.2526, 51.4044) centre (20.1404, 51.5167) ccw
  arc A1867 (19.5811, 51.7194) -> (19.6792, 52.0214) centre (19.6302, 51.8704) ccw
  line L563 (19.05, 51.9811) -> (19.05, 49.53)
  line L564 (19.1689, 51.9811) -> (19.05, 51.9811)
  arc A1868 (22.7022, 52.0786) -> (22.4777, 51.8541) centre (22.59, 51.9664) ccw
  line L565 (22.59, 51.9663) -> (21.9411, 52.2351)
  line L566 (19.6301, 51.8704) -> (19.4039, 51.9439)
  arc A1869 (27.3108, 51.0816) -> (27.4089, 50.7796) centre (27.3599, 50.9306) ccw
  arc A1870 (24.5123, 50.9143) -> (24.2878, 51.1388) centre (24.4001, 51.0266) ccw
  line L567 (24.0465, 50.673) -> (23.3553, 50.673)
  arc A1871 (28.2691, 50.8473) -> (28.3187, 51.1609) centre (28.2939, 51.0041) ccw
  line L568 (27.3599, 50.9306) -> (27.1479, 50.8226)
  line L569 (27.8211, 51.0413) -> (27.5861, 51.0041)
  line L570 (18.9311, 51.9811) -> (18.6961, 51.9439)
  arc A1872 (23.2332, 51.5305) -> (22.9399, 51.409) centre (23.0866, 51.4698) ccw
  arc A1873 (18.9311, 52.1398) -> (18.9311, 51.8223) centre (18.9311, 51.9811) ccw
  arc A1874 (21.2996, 52.0884) -> (21.1781, 52.3818) centre (21.2388, 52.2351) ccw
  arc A1875 (27.5613, 51.1609) -> (27.6109, 50.8473) centre (27.5861, 51.0041) ccw
  line L571 (19.8421, 51.7624) -> (19.6301, 51.8704)
  arc A1876 (27.8459, 50.8845) -> (27.7962, 51.1981) centre (27.821, 51.0413) ccw
  arc A1877 (18.7452, 51.7929) -> (18.647, 52.0949) centre (18.6961, 51.9439) ccw
  arc A1878 (19.9412, 51.4941) -> (20.1279, 51.751) centre (20.0346, 51.6226) ccw
  arc A1879 (19.05, 49.6888) -> (19.05, 49.3713) centre (19.05, 49.5301) ccw
  line L572 (28.5201, 50.9306) -> (28.2939, 51.0041)
  arc A1880 (29.4557, 50.4212) -> (29.1988, 50.6079) centre (29.3273, 50.5146) ccw
  line L573 (29.21, 50.3532) -> (29.0928, 50.5145)
  line L574 (18.6961, 51.9439) -> (18.4699, 51.8704)
  line L575 (18.4699, 51.8704) -> (18.2579, 51.7624)
  line L576 (18.2579, 51.7624) -> (18.0655, 51.6226)
  arc A1881 (23.514, 50.8209) -> (23.1965, 50.8209) centre (23.3553, 50.8209) ccw
  arc A1882 (22.5292, 51.8197) -> (22.6507, 52.113) centre (22.59, 51.9663) ccw
  line L577 (28.0589, 51.0413) -> (27.94, 51.0413)
  arc A1883 (28.8312, 50.5543) -> (29.0179, 50.8112) centre (28.9245, 50.6828) ccw
  line L578 (27.1479, 50.8226) -> (26.9555, 50.6828)
  line L579 (20.1404, 51.5167) -> (20.0345, 51.6226)
  arc A1884 (10.5423, 51.8541) -> (10.3178, 52.0786) centre (10.43, 51.9664) ccw
  line L580 (9.9335, 47.5902) -> (10.43, 47.0937)
  arc A1885 (10.0457, 47.7025) -> (9.8212, 47.478) centre (9.9335, 47.5903) ccw
  line L581 (10.43, 47.0937) -> (10.4521, 47.0845)
  line L582 (19.4039, 51.9439) -> (19.1689, 51.9811)
  arc A1886 (15.1277, 51.5841) -> (15.3523, 51.8086) centre (15.24, 51.6964) ccw
  arc A1887 (16.8611, 52.0763) -> (16.8611, 52.3938) centre (16.8611, 52.2351) ccw
  arc A1888 (18.6713, 52.1007) -> (18.7209, 51.7871) centre (18.6961, 51.9439) ccw
  arc A1889 (19.1938, 52.1379) -> (19.1441, 51.8243) centre (19.1689, 51.9811) ccw
  line L583 (21.2389, 52.2351) -> (20.59, 51.9663)
  line L584 (9.9335, 51.4698) -> (9.6647, 50.8209)
  line L585 (9.6647, 50.8209) -> (9.6647, 48.2391)
  arc A1890 (9.518, 50.8817) -> (9.8114, 50.7602) centre (9.6647, 50.821) ccw
  arc A1891 (16.1589, 52.3938) -> (16.1589, 52.0763) centre (16.1589, 52.2351) ccw
  arc A1892 (14.3211, 52.0763) -> (14.3211, 52.3938) centre (14.3211, 52.2351) ccw
  arc A1893 (10.3178, 46.9814) -> (10.5423, 47.2059) centre (10.43, 47.0936) ccw
  arc A1894 (19.7022, 52.0118) -> (19.5581, 51.7289) centre (19.6302, 51.8704) ccw
  arc A1895 (18.8912, 49.53) -> (19.2087, 49.53) centre (19.05, 49.53) ccw
  arc A1896 (18.3512, 51.6339) -> (18.1646, 51.8908) centre (18.2579, 51.7623) ccw
  arc A1897 (10.0801, 51.409) -> (9.7868, 51.5305) centre (9.9334, 51.4698) ccw
  line L586 (14.97, 51.9663) -> (14.3211, 52.2351)
  arc A1898 (24.0465, 50.5142) -> (24.0465, 50.8317) centre (24.0465, 50.673) ccw
  arc A1899 (9.8234, 50.8209) -> (9.506, 50.8209) centre (9.6647, 50.8209) ccw
  arc A1900 (10.3914, 46.9378) -> (10.5128, 47.2312) centre (10.4521, 47.0845) ccw
  arc A1901 (18.8913, 49.53) -> (19.2088, 49.53) centre (19.0501, 49.53) ccw
  line L587 (23.0865, 51.4698) -> (22.59, 51.9663)
  arc A1902 (19.3791, 51.7871) -> (19.4287, 52.1007) centre (19.4039, 51.9439) ccw
  arc A1903 (19.2088, 51.9811) -> (18.8913, 51.9811) centre (19.0501, 51.9811) ccw
  arc A1904 (23.2086, 50.7602) -> (23.502, 50.8817) centre (23.3553, 50.821) ccw
  arc A1905 (9.8114, 48.2998) -> (9.518, 48.1783) centre (9.6647, 48.239) ccw
  arc A1906 (19.9354, 51.8908) -> (19.7488, 51.6339) centre (19.8421, 51.7623) ccw
  line L588 (16.8611, 52.2351) -> (16.1589, 52.2351)
  arc A1907 (9.7868, 47.5295) -> (10.0801, 47.651) centre (9.9334, 47.5903) ccw
  arc A1908 (13.0823, 51.8541) -> (12.8578, 52.0786) centre (12.9701, 51.9664) ccw
  arc A1909 (13.6189, 52.3938) -> (13.6189, 52.0763) centre (13.6189, 52.2351) ccw
  line L589 (19.05, 51.9811) -> (18.9311, 51.9811)
  arc A1910 (11.1396, 52.0884) -> (11.0181, 52.3818) centre (11.0788, 52.2351) ccw
  arc A1911 (19.77, 51.6209) -> (19.9142, 51.9038) centre (19.8421, 51.7623) ccw
  arc A1912 (19.453, 52.0949) -> (19.3548, 51.7929) centre (19.4039, 51.9439) ccw
  line L590 (9.6647, 48.2391) -> (9.9335, 47.5902)
  arc A1913 (20.0281, 51.4044) -> (20.2526, 51.629) centre (20.1403, 51.5167) ccw
  arc A1914 (16.2196, 52.0884) -> (16.0981, 52.3818) centre (16.1589, 52.2351) ccw
  line L591 (15.24, 51.6963) -> (14.97, 51.9663)
  arc A1915 (12.3692, 51.8197) -> (12.4907, 52.113) centre (12.43, 51.9663) ccw
  arc A1916 (17.4492, 51.8197) -> (17.5707, 52.113) centre (17.51, 51.9663) ccw
  arc A1917 (22.9743, 51.3575) -> (23.1988, 51.582) centre (23.0865, 51.4698) ccw
  arc A1918 (9.8212, 51.582) -> (10.0457, 51.3575) centre (9.9335, 51.4698) ccw
  arc A1919 (11.8419, 52.3818) -> (11.7204, 52.0884) centre (11.7812, 52.2351) ccw
  line L592 (12.7, 51.6963) -> (12.43, 51.9663)
  arc A1920 (19.05, 51.8223) -> (19.05, 52.1398) centre (19.05, 51.9811) ccw
  arc A1921 (16.9219, 52.3818) -> (16.8004, 52.0884) centre (16.8612, 52.2351) ccw
  line L593 (10.43, 51.9663) -> (9.9335, 51.4698)
  line L594 (20.59, 51.9663) -> (20.1404, 51.5167)
  line L595 (18.0655, 51.6226) -> (17.9596, 51.5167)
  arc A1922 (9.506, 48.2391) -> (9.8234, 48.2391) centre (9.6647, 48.2391) ccw
  arc A1923 (17.9721, 51.751) -> (18.1588, 51.4941) centre (18.0654, 51.6226) ccw
  line L596 (17.51, 51.9663) -> (16.8611, 52.2351)
  arc A1924 (15.6223, 51.8541) -> (15.3978, 52.0786) centre (15.51, 51.9664) ccw
  arc A1925 (15.4493, 52.113) -> (15.5708, 51.8197) centre (15.5101, 51.9664) ccw
  arc A1926 (11.7811, 52.0763) -> (11.7811, 52.3938) centre (11.7811, 52.2351) ccw
  arc A1927 (13.6796, 52.0884) -> (13.5581, 52.3818) centre (13.6189, 52.2351) ccw
  arc A1928 (19.1689, 51.8223) -> (19.1689, 52.1398) centre (19.1689, 51.9811) ccw